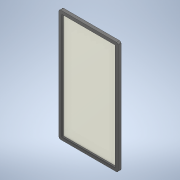
# Autodesk Inventor part: Tavla 35x70
Saved by Autodesk Inventor 2020 (Build 240168000, 168)
## iProperties
Created: 2020-02-29
Part Number: Tavla 35x70
Material: Generic
Document SubType Name: Modeling
Designer: Patrik
Density: 1 g/cm^3
Appearance: Smooth - Black
Author: Patrik
Autodesk Inventor part; units mm, degrees
ref_plane "YZ Plane" through (0, 0, 0) normal (1, 0, 0) x (0, 1, 0)
ref_plane "XZ Plane" through (0, 0, 0) normal (0, 1, 0) x (-1, 0, 0)
ref_plane "XY Plane" through (0, 0, 0) normal (0, 0, 1) x (1, 0, 0)
sketch "Sketch1" plane through (0, 0, 0) normal (0, 0, 1) x (1, 0, 0)
  line L0 (0, 0) -> (390, 0)
  line L1 (390, 0) -> (390, 740)
  line L2 (390, 740) -> (0, 740)
  line L3 (0, 740) -> (0, 0)
  dimension "d0" = 390
  dimension "d1" = 740
  constraints: 8 end point, 2 parallel, 1 horizontal, 1 perpendicular
  measures "d0" distance of L2.end L1.end
  measures "d1" distance of L1.end L0.end
extrude "Extrusion1" add sketch "Sketch1" along normal blind 20
sketch "Sketch2" plane through (0, 0, 20) normal (0, 0, 1) x (1, 0, 0)
  line L0 (20, 20) -> (370, 20)
  line L1 (370, 20) -> (370, 720)
  line L2 (370, 720) -> (20, 720)
  line L3 (20, 720) -> (20, 20)
  point P0 (0, 0)
  dimension "d6" = 350
  dimension "d7" = 700
  constraints: 8 end point, 2 parallel, 1 horizontal, 1 perpendicular
  measures "d6" distance of L2.end L1.end
  measures "d7" distance of L1.end L0.end
extrude "Extrusion2" cut sketch "Sketch2" against normal blind 10
fillet "Fillet1" radius 10 4 edges at (390, 740, 10) (390, 0, 10) (0, 740, 10) (0, 0, 10)
body "Solid1"
